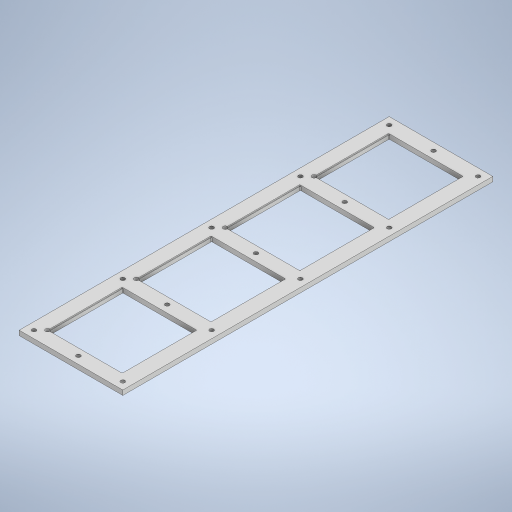
# Autodesk Inventor part: BBM Jig
Saved by Autodesk Inventor 2023 (Build 270158000, 158)
## iProperties
Created: 2022-10-25
Part Number: BBM Jig
Material: Generic
Document SubType Name: Modeling
Designer: Caleb
Density: 1 g/cm^3
Appearance: Default
Author: Caleb
Autodesk Inventor part; units mm, degrees
ref_plane "YZ Plane" through (0, 0, 0) normal (1, 0, 0) x (0, 1, 0)
ref_plane "XZ Plane" through (0, 0, 0) normal (0, 1, 0) x (-1, 0, 0)
ref_plane "XY Plane" through (0, 0, 0) normal (0, 0, 1) x (1, 0, 0)
sketch "Sketch1" plane through (0, 0, 0) normal (0, 1, 0) x (-1, 0, 0)
  line L0 (-17.5, -62.5) -> (17.5, -62.5)
  line L1 (17.5, -62.5) -> (17.5, 62.5)
  line L2 (17.5, 62.5) -> (-17.5, 62.5)
  line L3 (-17.5, 62.5) -> (-17.5, -62.5)
  line L4 (-17.5, -62.5) -> (17.5, 62.5) construction
  line L5 (17.5, -62.5) -> (-17.5, 62.5) construction
  point P0 (0, 0)
  dimension "d0" = 35
  dimension "d1" = 125
  constraints: 12 end point, 2 midpoint, 2 parallel, 1 horizontal, 1 perpendicular
  measures "d0" distance of L2.end L1.end
  measures "d1" distance of L1.end L0.end
extrude "Extrusion1" add sketch "Sketch1" along normal blind 1.5875
sketch "Sketch2" plane through (0, 1.5875, 0) normal (0, 1, 0) x (1, 0, 0)
  line L0 (-12.25, -57.5) -> (12.25, -57.5)
  line L1 (12.5, -57.25) -> (12.5, -32.75)
  line L2 (12.25, -32.5) -> (-12.25, -32.5)
  line L3 (-12.5, -32.75) -> (-12.5, -57.25)
  line L4 (-17.5, -62.5) -> (17.5, -62.5) projected
  line L5 (-17.5, 62.5) -> (-17.5, -62.5) projected
  arc A0 (-12.25, -32.5) -> (-12.5, -32.75) centre (-12.25, -32.75) ccw
  arc A1 (12.5, -32.75) -> (12.25, -32.5) centre (12.25, -32.75) ccw
  arc A2 (12.25, -57.5) -> (12.5, -57.25) centre (12.25, -57.25) ccw
  arc A3 (-12.5, -57.25) -> (-12.25, -57.5) centre (-12.25, -57.25) ccw
  arc A4 (-12.5, -27.25) -> (-12.25, -27.5) centre (-12.25, -27.25) ccw
  line L6 (-12.25, -27.5) -> (12.25, -27.5)
  arc A5 (12.25, -27.5) -> (12.5, -27.25) centre (12.25, -27.25) ccw
  line L7 (-12.5, -2.75) -> (-12.5, -27.25)
  arc A6 (-12.25, -2.5) -> (-12.5, -2.75) centre (-12.25, -2.75) ccw
  line L8 (12.5, -27.25) -> (12.5, -2.75)
  line L9 (12.25, -2.5) -> (-12.25, -2.5)
  arc A7 (12.5, -2.75) -> (12.25, -2.5) centre (12.25, -2.75) ccw
  arc A8 (-12.5, 2.75) -> (-12.25, 2.5) centre (-12.25, 2.75) ccw
  line L10 (-12.25, 2.5) -> (12.25, 2.5)
  arc A9 (12.25, 2.5) -> (12.5, 2.75) centre (12.25, 2.75) ccw
  line L11 (-12.5, 27.25) -> (-12.5, 2.75)
  arc A10 (-12.25, 27.5) -> (-12.5, 27.25) centre (-12.25, 27.25) ccw
  line L12 (12.5, 2.75) -> (12.5, 27.25)
  line L13 (12.25, 27.5) -> (-12.25, 27.5)
  arc A11 (12.5, 27.25) -> (12.25, 27.5) centre (12.25, 27.25) ccw
  arc A12 (-12.5, 32.75) -> (-12.25, 32.5) centre (-12.25, 32.75) ccw
  line L14 (-12.25, 32.5) -> (12.25, 32.5)
  arc A13 (12.25, 32.5) -> (12.5, 32.75) centre (12.25, 32.75) ccw
  line L15 (-12.5, 57.25) -> (-12.5, 32.75)
  arc A14 (-12.25, 57.5) -> (-12.5, 57.25) centre (-12.25, 57.25) ccw
  line L16 (12.5, 32.75) -> (12.5, 57.25)
  line L17 (12.25, 57.5) -> (-12.25, 57.5)
  arc A15 (12.5, 57.25) -> (12.25, 57.5) centre (12.25, 57.25) ccw
  point P0 (0, 0)
  point P1 (-12.5, -57.5)
  point P2 (12.5, -32.5)
  point P3 (12.5, -57.5)
  point P4 (-12.5, -32.5)
  point P5 (12.5, -27.5)
  point P6 (-12.5, -27.5)
  point P7 (-12.5, -2.5)
  point P8 (12.5, -2.5)
  point P9 (12.5, 2.5)
  point P10 (-12.5, 2.5)
  point P11 (-12.5, 27.5)
  point P12 (12.5, 27.5)
  point P13 (12.5, 32.5)
  point P14 (-12.5, 32.5)
  point P15 (-12.5, 57.5)
  point P16 (12.5, 57.5)
  dimension "d4" = 5
  dimension "d5" = 5
  dimension "d6" = 25
  dimension "d7" = 25
  dimension "d18" = 0.25
  dimension "d21" = 30
  constraints: 32 end point, 32 point on circle, 32 point on line, 16 centre point, 8 tangent, 3 equal radius, 2 parallel, 1 horizontal, 1 perpendicular, 1 vertical, 72 other
  measures "d4" distance between parallel lines of L4 L0
  measures "d5" distance between parallel lines of L5 L3
  measures "d6" distance of point (-12.5, -32.5) point (-12.5, -57.5)
  measures "d7" distance of point (12.5, -32.5) point (-12.5, -32.5)
  measures "d18" radius of A0
  measures "d21" distance of L3.end L7.end
extrude "Extrusion2" cut sketch "Sketch2" against normal through all
sketch "Sketch3" plane through (0, 1.5875, 0) normal (0, 1, 0) x (1, 0, 0)
  line L0 (-12.5, -57.25) -> (-12.5, -32.75) projected
  line L1 (-12.5, -32.5) -> (-12.45, -32.5)
  line L2 (-12.7, -32.75) -> (-12.7, -57.7)
  line L3 (-12.7, -57.7) -> (12.25, -57.7)
  line L4 (12.25, -57.5) -> (-12.25, -57.5) projected
  line L5 (-12.25, -32.5) -> (12.25, -32.5) projected
  arc A0 (-12.25, -32.5) -> (-12.5, -32.75) centre (-12.25, -32.75) ccw projected
  line L6 (-12.5, -32.5) -> (-12.25, -32.5)
  arc A1 (12.25, -57.5) -> (12.5, -57.25) centre (12.25, -57.25) ccw projected
  line L7 (12.5, -57.45) -> (12.5, -57.25)
  arc A2 (12.25, -57.7) -> (12.5, -57.45) centre (12.25, -57.45) ccw
  arc A3 (-12.45, -32.5) -> (-12.7, -32.75) centre (-12.45, -32.75) ccw
  line L8 (12.5, -32.75) -> (12.5, -57.25) projected
  arc A4 (12.5, -32.75) -> (12.25, -32.5) centre (12.25, -32.75) ccw projected
  arc A5 (-12.5, -57.25) -> (-12.25, -57.5) centre (-12.25, -57.25) ccw projected
  line L9 (-12.5, -2.5) -> (-12.45, -2.5)
  line L10 (-12.5, -2.5) -> (-12.25, -2.5)
  arc A6 (-12.45, -2.5) -> (-12.7, -2.75) centre (-12.45, -2.75) ccw
  line L11 (-12.7, -2.75) -> (-12.7, -27.7)
  line L12 (-12.7, -27.7) -> (12.25, -27.7)
  line L13 (12.5, -27.45) -> (12.5, -27.25)
  arc A7 (12.25, -27.7) -> (12.5, -27.45) centre (12.25, -27.45) ccw
  line L14 (-12.5, 27.5) -> (-12.45, 27.5)
  line L15 (-12.5, 27.5) -> (-12.25, 27.5)
  arc A8 (-12.45, 27.5) -> (-12.7, 27.25) centre (-12.45, 27.25) ccw
  line L16 (-12.7, 27.25) -> (-12.7, 2.3)
  line L17 (-12.7, 2.3) -> (12.25, 2.3)
  line L18 (12.5, 2.55) -> (12.5, 2.75)
  arc A9 (12.25, 2.3) -> (12.5, 2.55) centre (12.25, 2.55) ccw
  line L19 (-12.5, 57.5) -> (-12.45, 57.5)
  line L20 (-12.5, 57.5) -> (-12.25, 57.5)
  arc A10 (-12.45, 57.5) -> (-12.7, 57.25) centre (-12.45, 57.25) ccw
  line L21 (-12.7, 57.25) -> (-12.7, 32.3)
  line L22 (-12.7, 32.3) -> (12.25, 32.3)
  line L23 (12.5, 32.55) -> (12.5, 32.75)
  arc A11 (12.25, 32.3) -> (12.5, 32.55) centre (12.25, 32.55) ccw
  arc A12 (12.25, 32.5) -> (12.5, 32.75) centre (12.25, 32.75) ccw projected
  line L24 (12.25, 32.5) -> (-12.25, 32.5) projected
  arc A13 (-12.5, 32.75) -> (-12.25, 32.5) centre (-12.25, 32.75) ccw projected
  line L25 (-12.5, 32.75) -> (-12.5, 57.25) projected
  arc A14 (-12.25, 57.5) -> (-12.5, 57.25) centre (-12.25, 57.25) ccw projected
  line L26 (-12.25, 57.5) -> (12.25, 57.5) projected
  arc A15 (12.5, 57.25) -> (12.25, 57.5) centre (12.25, 57.25) ccw projected
  line L27 (12.5, 57.25) -> (12.5, 32.75) projected
  arc A16 (12.25, 2.5) -> (12.5, 2.75) centre (12.25, 2.75) ccw projected
  line L28 (12.25, 2.5) -> (-12.25, 2.5) projected
  arc A17 (-12.5, 2.75) -> (-12.25, 2.5) centre (-12.25, 2.75) ccw projected
  line L29 (-12.5, 2.75) -> (-12.5, 27.25) projected
  arc A18 (-12.25, 27.5) -> (-12.5, 27.25) centre (-12.25, 27.25) ccw projected
  line L30 (-12.25, 27.5) -> (12.25, 27.5) projected
  arc A19 (12.5, 27.25) -> (12.25, 27.5) centre (12.25, 27.25) ccw projected
  line L31 (12.5, 27.25) -> (12.5, 2.75) projected
  arc A20 (-12.5, -57.25) -> (-12.25, -57.5) centre (-12.25, -57.25) ccw projected
  line L32 (-12.5, -57.25) -> (-12.5, -32.75) projected
  arc A21 (-12.25, -32.5) -> (-12.5, -32.75) centre (-12.25, -32.75) ccw projected
  line L33 (-12.25, -32.5) -> (12.25, -32.5) projected
  arc A22 (12.5, -32.75) -> (12.25, -32.5) centre (12.25, -32.75) ccw projected
  line L34 (12.5, -32.75) -> (12.5, -57.25) projected
  arc A23 (12.25, -57.5) -> (12.5, -57.25) centre (12.25, -57.25) ccw projected
  line L35 (12.25, -57.5) -> (-12.25, -57.5) projected
  arc A24 (12.25, -27.5) -> (12.5, -27.25) centre (12.25, -27.25) ccw projected
  line L36 (12.25, -27.5) -> (-12.25, -27.5) projected
  arc A25 (-12.5, -27.25) -> (-12.25, -27.5) centre (-12.25, -27.25) ccw projected
  line L37 (-12.5, -27.25) -> (-12.5, -2.75) projected
  arc A26 (-12.25, -2.5) -> (-12.5, -2.75) centre (-12.25, -2.75) ccw projected
  line L38 (-12.25, -2.5) -> (12.25, -2.5) projected
  arc A27 (12.5, -2.75) -> (12.25, -2.5) centre (12.25, -2.75) ccw projected
  line L39 (12.5, -2.75) -> (12.5, -27.25) projected
  line L40 (-17.5, 62.5) -> (-17.5, -62.5) projected
  line L41 (-17.5, -62.5) -> (17.5, -62.5) projected
  line L42 (17.5, -62.5) -> (17.5, 62.5) projected
  line L43 (17.5, 62.5) -> (-17.5, 62.5) projected
  point P0 (0, 0)
  point P1 (-12.5, -45.8)
  point P2 (-12.7, -32.5)
  point P3 (12.5, -57.7)
  point P4 (12.5, -20.8)
  point P5 (12.5, -45.8)
  point P6 (-12.7, -2.5)
  point P7 (12.5, -2.75)
  point P8 (12.25, -2.75)
  point P9 (12.25, -2.5)
  point P10 (-12.25, -2.75)
  point P11 (-12.5, -2.75)
  point P12 (-12.5, -15.8)
  point P13 (12.5, -15.8)
  point P14 (-12.5, -27.25)
  point P15 (-12.25, -27.25)
  point P16 (12.5, -27.7)
  point P17 (-12.25, -27.5)
  point P18 (12.25, -27.25)
  point P19 (12.25, -27.5)
  point P20 (-12.7, 27.5)
  point P21 (12.5, 27.25)
  point P22 (12.25, 27.25)
  point P23 (12.25, 27.5)
  point P24 (-12.25, 27.25)
  point P25 (-12.5, 27.25)
  point P26 (-12.5, 14.2)
  point P27 (12.5, 14.2)
  point P28 (-12.5, 2.75)
  point P29 (-12.25, 2.75)
  point P30 (12.5, 2.3)
  point P31 (-12.25, 2.5)
  point P32 (12.25, 2.75)
  point P33 (12.25, 2.5)
  point P34 (-12.7, 57.5)
  point P35 (12.5, 57.25)
  point P36 (12.25, 57.25)
  point P37 (12.25, 57.5)
  point P38 (-12.25, 57.25)
  point P39 (-12.5, 57.25)
  point P40 (-12.5, 44.2)
  point P41 (12.5, 44.2)
  point P42 (-12.5, 32.75)
  point P43 (-12.25, 32.75)
  point P44 (12.5, 32.3)
  point P45 (-12.25, 32.5)
  point P46 (12.25, 32.75)
  point P47 (12.25, 32.5)
  point P48 (12.5, 32.75)
  point P49 (12.5, 2.75)
  point P50 (-12.25, 27.5)
  point P51 (12.5, -27.25)
  point P52 (-12.25, -2.5)
  dimension "d11" = 25.2
  dimension "d26" = 0.25
  dimension "d29" = 30
  dimension "d42" = 0.2
  constraints: 40 end point, 16 point on circle, 16 point on line, 8 centre point, 6 tangent, 3 horizontal, 2 vertical, 1 equal radius, 1 horizontal alignment, 1 perpendicular, 1 vertical alignment, 94 other
  measures "d11" distance of point (-12.7, -32.5) L2.end
  measures "d26" radius of A2
  measures "d29" distance of L1.start L9.start
  measures "d42" distance between parallel lines of L2 L0
extrude "Extrusion3" cut sketch "Sketch3" against normal blind 0.35 contours A5 L4 A1 L7 A2 L3 L2 A3 L6 A0 L0 | L10 A26 L37 A25 L36 A24 L13 A7 L12 L11 A6 | L15 A18 L29 A17 L28 A16 L18 A9 L17 L16 A8 | L20 A14 L25 A13 L24 A12 L23 A11 L22 L21 A10
sketch "Sketch4" plane through (0, 1.5875, 0) normal (0, 1, 0) x (1, 0, 0)
  line L0 (-12.7, -57.7) -> (-12.7, -32.75) projected
  line L1 (-12.7, -57.7) -> (-12.7, -32.75) projected
  circle A0 centre (-12.7, -57.7) radius 0.75
  circle A1 centre (-12.7, -27.7) radius 0.75
  circle A2 centre (-12.7, 2.3) radius 0.75
  circle A3 centre (-12.7, 32.3) radius 0.75
  point P0 (0, 0)
  dimension "d34" = 1.5
  dimension "d37" = 30
  constraints: 4 centre point, 1 coincident, 1 vertical, 6 other
  measures "d34" diameter of A0
  measures "d37" distance of A0.centre A1.centre
extrude "Extrusion4" cut sketch "Sketch4" against normal through all
sketch "Sketch5" plane through (0, 0, 0) normal (0, -1, 0) x (1, 0, 0)
  line L0 (-17.5, 62.5) -> (17.5, 62.5) projected
  line L1 (17.5, 62.5) -> (17.5, -62.5) projected
  line L2 (-17.5, -62.5) -> (-17.5, 62.5) projected
  point P0 (0, 0)
  point P1 (15, 60)
  point P2 (0, 60)
  point P3 (-15, 60)
  point P4 (-15, 30)
  point P5 (0, 30)
  point P6 (15, 30)
  point P7 (-15, 0)
  point P8 (0, 0)
  point P9 (15, 0)
  point P10 (-15, -30)
  point P11 (0, -30)
  point P12 (15, -30)
  point P13 (-15, -60)
  point P14 (0, -60)
  point P15 (15, -60)
  dimension "d43" = 2.5
  dimension "d44" = 2.5
  dimension "d45" = 2.5
  dimension "d48" = 30
  constraints: 2 horizontal alignment, 1 vertical, 1 vertical alignment, 12 other
  measures "d43" distance from line of L0 point (15, 60)
  measures "d44" distance from line of L1 point (15, 60)
  measures "d45" distance from line of L2 point (-15, 60)
  measures "d48" distance of point (-15, 60) point (-15, 30)
hole "Hole1" at (15, 0, 60) at (0, 0, 60) at (-15, 0, 60) at (-15, 0, 30) at (0, 0, 30) at (15, 0, 30) at (-15, 0, 0) at (0, 0, 0) at (15, 0, 0) at (-15, 0, -30) at (0, 0, -30) at (15, 0, -30) at (-15, 0, -60) at (0, 0, -60) at (15, 0, -60) direction (0, 1, 0) diameter 1.4249 end through all thread size "1-64 UNC" class "2B" standard "ANSI Unified Screw Threads"
body "Solid1"
